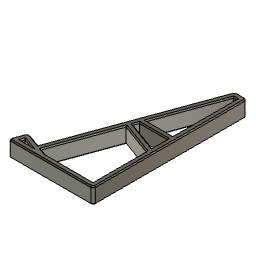
3D Printable Stand v1.0 - Large (Autodesk Fusion 360 design; units mm, degrees)
Autodesk Fusion 360 part; units mm, degrees
sketch "Sketch1" plane through (0, 0, 0) normal (0, 0, 1) x (1, 0, 0)
  line L0 (0, 0) -> (5.1303, 14.0954)
  line L1 (0, 0) -> (15, 0) construction
  line L2 (5.1303, 14.0954) -> (19.2257, 8.9651)
  line L3 (5.1303, 14.0954) -> (20.1303, 14.0954) construction
  line L4 (19.2257, 8.9651) -> (99.2257, 8.9651) construction
  line L5 (46.5873, 84.1405) -> (55, 84.1405)
  line L6 (80, 145) -> (80, 0)
  line L7 (0, 0) -> (80, 0)
  line L8 (19.2257, 8.9651) -> (68.7384, 145)
  line L9 (19.2257, 8.9651) -> (163.991, 8.9651) construction
  line L10 (68.7384, 145) -> (80, 145)
  dimension "d1" = 70
  dimension "d2" = 15
  dimension "d3" = 20
  dimension "d4" = 15
  dimension "d6" = 80
  dimension "d52" = 70
  constraint horizontal L1
  constraint coincident L0.start L1.start
  constraint horizontal L3
  constraint horizontal L4
  constraint horizontal L5
  constraint perpendicular L4 L6
  constraint perpendicular L6 L7
  constraint horizontal L9
  constraint perpendicular L6 L10
  measures "d1" angle of L0 L1
  measures "d2" distance of L0.start L0.end
  measures "d3" angle of L2 L3
  measures "d4" distance of L0.end L2.end
  measures "d6" distance of L2.end L5.start
  measures "d52" angle of L8 L9
extrude "Extrude1" add sketch "Sketch1" along normal blind 15
sketch "Sketch2" plane through (0, 0, 15) normal (0, 0, 1) x (-1, 0, 0)
  line L0 (-19.2257, -8.9651) -> (-5.1303, -14.0954)
  line L1 (-5.1303, -14.0954) -> (0, 0)
  line L2 (-23.9242, -7.255) -> (52.1783, -7.255) construction
  line L3 (-23.9242, -7.255) -> (-30.1197, -5)
  line L4 (-23.9242, -7.255) -> (-17.331, -7.255) construction
  line L5 (0, 0) -> (-80, 0)
  line L6 (-80, 0) -> (-80, -145)
  line L7 (-80, -145) -> (-68.7384, -145)
  line L8 (-68.7384, -145) -> (-19.2257, -8.9651)
  line L9 (-30.1197, -5) -> (-75, -5)
  line L10 (-23.9242, -7.255) -> (117.3401, -7.255) construction
  line L11 (-72.2394, -140) -> (-75, -140)
  line L12 (-75, -55) -> (-45.2438, -65.8304)
  line L13 (-75, -60.3209) -> (-46.9539, -70.5288)
  line L14 (-75, -75) -> (-48.5813, -75)
  line L15 (-75, -80) -> (-50.4012, -80)
  line L16 (-75, -140) -> (-75, -80)
  line L17 (-75, -60.3209) -> (-75, -75)
  line L18 (-75, -55) -> (-75, -5)
  line L19 (-72.2394, -140) -> (-50.4012, -80)
  line L20 (-48.5813, -75) -> (-46.9539, -70.5288)
  line L21 (-45.2438, -65.8304) -> (-23.9242, -7.255)
  dimension "d13" = 5
  dimension "d15" = 160
  constraint horizontal L2
  constraint horizontal L4
  constraint horizontal L9
  constraint horizontal L10
  constraint perpendicular L15 L16
  constraint perpendicular L14 L17
  constraint perpendicular L9 L18
  constraint perpendicular L13 L20
  constraint perpendicular L3 L21
  measures "d13" distance of L0.start L2.start
  measures "d15" angle of L3 L4
extrude "Extrude2" cut sketch "Sketch2" against normal blind 78 contours L3 L9 L12 L18 L21
sketch "Sketch3" plane through (0, 0, 15) normal (0, 0, 1) x (-1, 0, 0)
  line L0 (-30.1197, -5) -> (-23.9242, -7.255)
  line L1 (-19.2257, -8.9651) -> (-5.1303, -14.0954)
  line L2 (-5.1303, -14.0954) -> (0, 0)
  line L3 (-7.1358, -4.9864) -> (-15.5382, -4.9864)
  line L4 (-7.1358, -4.9864) -> (-8.1187, -7.6868)
  line L5 (-8.1187, -7.6868) -> (-15.5382, -4.9864)
  line L6 (0, 0) -> (-80, 0)
  line L7 (-80, 0) -> (-80, -145)
  line L8 (-80, -145) -> (-68.7384, -145)
  line L9 (-68.7384, -145) -> (-19.2257, -8.9651)
  line L10 (-75, -5) -> (-30.1197, -5)
  line L11 (-23.9242, -7.255) -> (-45.2438, -65.8304)
  line L12 (-45.2438, -65.8304) -> (-75, -55)
  line L13 (-75, -55) -> (-75, -5)
  constraint perpendicular L4 L5
extrude "Extrude3" cut sketch "Sketch3" against normal blind 57 contours L3 L4 L5
extrude "Extrude7" cut sketch "Sketch2" against normal blind 27 contours L13 L14 L17 L20
extrude "Extrude8" cut sketch "Sketch2" against normal blind 32 contours L11 L15 L16 L19
chamfer "Chamfer18" distance 2 angle 45 2 edges at (5.1303, 14.0954, 7.5) (0, 0, 7.5)
chamfer "Chamfer19" distance 2 angle 45 1 edges at (80, 0, 7.5)
chamfer "Chamfer20" distance 2 angle 45 2 edges at (80, 145, 7.5) (68.7384, 145, 7.5)
chamfer "Chamfer21" distance 1 angle 45 27 edges at (43.64, 76.0429, 15) (13.1177, 11.1882, 15) (5.728, 12.8137, 15) (2.5652, 7.0477, 15) (1.342, 0.9397, 15) (40, 0, 15) (11.337, 4.9864, 15) (7.6272, 6.3366, 15) (11.8284, 6.3366, 15) (27.0219, 6.1275, 15) (52.5598, 5, 15) (34.584, 36.5427, 15) (75, 30, 15) (79, 1, 15) (80, 72.5, 15) (60.1219, 60.4152, 15) (60.977, 65.4249, 15) (75, 67.6604, 15) (61.7907, 75, 15) (47.7676, 72.7644, 15) (61.3203, 110, 15) (62.7006, 80, 15) (75, 110, 15) (79, 144, 15) (74.3692, 145, 15) (69.3963, 144.0603, 15) (73.6197, 140, 15)
chamfer "Chamfer22" distance 1 angle 45 27 edges at (40, 0, 0) (1.342, 0.9397, 0) (2.5652, 7.0477, 0) (5.728, 12.8137, 0) (13.1177, 11.1882, 0) (11.8284, 6.3366, 0) (7.6272, 6.3366, 0) (11.337, 4.9864, 0) (27.0219, 6.1275, 0) (52.5598, 5, 0) (79, 1, 0) (80, 72.5, 0) (75, 30, 0) (34.584, 36.5427, 0) (43.64, 76.0429, 0) (60.1219, 60.4152, 0) (60.977, 65.4249, 0) (75, 67.6604, 0) (61.7907, 75, 0) (47.7676, 72.7644, 0) (61.3203, 110, 0) (62.7006, 80, 0) (75, 110, 0) (73.6197, 140, 0) (69.3963, 144.0603, 0) (74.3692, 145, 0) (79, 144, 0)
extrude "Extrude6" [rolled back] along distance -20 taper angle 0
